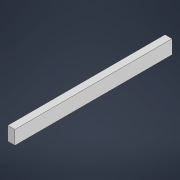
# Autodesk Inventor part: Sliding Pin
Saved by Autodesk Inventor 2022 (Build 260153000, 153)
## iProperties
Created: 2021-06-04
Part Number: Sliding Pin
Material: Generic
Document SubType Name: Modeling
Designer: saatvik123
Density: 1 g/cm^3
Appearance: Default
Author: saatvik123
## iProperties of the stored document Sliding Pin_3DPrint.ipt
Created: 2021-06-06
Part Number: Sliding Pin_3DPrint
Material: Generic
Document SubType Name: Modeling
Designer: sidsa
Density: 1 g/cm^3
Appearance: Default
Author: sidsa
Autodesk Inventor part; units mm, degrees
ref_plane "YZ Plane" through (0, 0, 0) normal (1, 0, 0) x (0, 1, 0)
ref_plane "XZ Plane" through (0, 0, 0) normal (0, 1, 0) x (-1, 0, 0)
ref_plane "XY Plane" through (0, 0, 0) normal (0, 0, 1) x (1, 0, 0)
sketch "Sketch1" plane through (0, 0, 0) normal (0, 0, 1) x (1, 0, 0)
  line L0 (-22.225, -2.3815) -> (-24.765, -2.3815) projected
  line L1 (-22.225, 2.3375) -> (-22.225, -2.3815) projected
  line L2 (-24.765, 2.3375) -> (-22.225, 2.3375) projected
  line L3 (-24.765, -2.3815) -> (-24.765, 2.3375) projected
  line L4 (-24.638, -2.2545) -> (-22.352, -2.2545)
  line L5 (-22.352, -2.2545) -> (-22.352, 2.2105)
  line L6 (-22.352, 2.2105) -> (-24.638, 2.2105)
  line L7 (-24.638, 2.2105) -> (-24.638, -2.2545)
  point P0 (0, 0)
  dimension "d0" = 0.127
  constraints: 8 end point, 3 other
  measures "d0" distance between parallel lines of L0 L4
extrude "Extrusion1" add sketch "Sketch1" along normal blind 50.8 contours L7 L6 L5 L4
body "Solid1"
